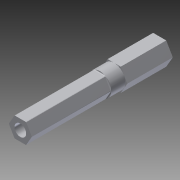
# Autodesk Inventor part: Base OutputShaft
Saved by Autodesk Inventor 2013 (Build 170138000, 138)
## iProperties
Created: 2013-06-25
Part Number: Base OutputShaft
Material: Generic
Document SubType Name: Modeling
Designer: mvarma
Density: 1 g/cm^3
Author: mvarma
Autodesk Inventor part; units mm, degrees
ref_plane "YZ Plane" through (0, 0, 0) normal (1, 0, 0) x (0, 1, 0)
ref_plane "XZ Plane" through (0, 0, 0) normal (0, 1, 0) x (-1, 0, 0)
sketch "Sketch1" plane through (0, 0, 0) normal (0, 0, 1) x (1, 0, 0)
  line L0 (-7.3323, 0) -> (-3.6662, 6.35)
  line L1 (-3.6662, 6.35) -> (3.6662, 6.35)
  line L2 (3.6662, 6.35) -> (7.3323, 0)
  line L3 (7.3323, 0) -> (3.6662, -6.35)
  line L4 (3.6662, -6.35) -> (-3.6662, -6.35)
  line L5 (-3.6662, -6.35) -> (-7.3323, 0)
  point P0 (0, 0)
  point P1 (0, 0)
  dimension "d0" = 12.7
  constraints: 12 end point, 1 coincident, 1 horizontal, 13 other
  measures "d0" distance between parallel lines of L4 L1
extrude "Extrusion1" add sketch "Sketch1" along normal blind 25.4
sketch "Sketch2" plane through (0, 0, 25.4) normal (0, 0, 1) x (1, 0, 0)
  circle A0 centre (0, 0) radius 6.35
  circle A1 centre (0, 0) radius 7.9375
  dimension "d3" = 12.7
  dimension "d18" = 15.875
  constraints: 2 centre point, 2 coincident
  measures "d3" diameter of A0
  measures "d18" diameter of A1
extrude "Extrusion2" add sketch "Sketch2" along normal blind 7.9375 contours A0
ref_plane "Work Plane1" through (0, 0, 33.3375) normal (0, 0, 1) x (1, 0, 0)
sketch "Sketch3" plane through (0, 0, 33.3375) normal (0, 0, 1) x (1, 0, 0)
  circle A0 centre (0, 0) radius 6.35 projected
  line L0 (-6.4158, 0) -> (-3.2079, 5.5562)
  line L1 (-3.2079, 5.5562) -> (3.2079, 5.5563)
  line L2 (3.2079, 5.5563) -> (6.4158, 0)
  line L3 (6.4158, 0) -> (3.2079, -5.5563)
  line L4 (3.2079, -5.5563) -> (-3.2079, -5.5563)
  line L5 (-3.2079, -5.5563) -> (-6.4158, 0)
  dimension "d7" = 11.1125
  constraints: 12 end point, 1 coincident, 1 horizontal, 13 other
  measures "d7" distance between parallel lines of L4 L1
extrude "Extrusion3" add sketch "Sketch3" along normal blind 44.45 contours A0 L3 L4 L5 L0 L1 L2 | A0 L2 L3 | A0 L1 L2 | L3 L4 A0 | A0 L0 L1 | L4 L5 A0 | A0 L5 L0
extrude "Extrusion6" cut sketch "Sketch2" along normal through all
fillet "Fillet1" radius 0.508 6 edges at (0, 5.5562, 33.3375) (4.8119, 2.7781, 33.3375) (4.8119, -2.7781, 33.3375) (0, -5.5563, 33.3375) (-4.8119, -2.7781, 33.3375) (-4.8119, 2.7781, 33.3375)
sketch "Sketch6" plane through (0, 0, 77.7875) normal (0, 0, 1) x (1, 0, 0)
  arc A0 (-3.0742, 5.5562) -> (-3.2748, 5.4404) centre (0, 0) ccw projected
  constraints: 1 coincident
hole "Hole2" at (0, 0, 77.7875) direction (0, 0, -1) diameter 6.5278 end through all clearance for "Socket Head Cap Screw" size "1/4" standard "Ansi Unified Screw Threads"
body "Solid1"
